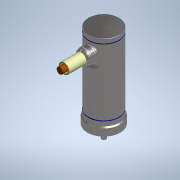
# Autodesk Inventor part: AKMH23x-CCTNCAFK
Saved by Autodesk Inventor 2021 (Build 250183000, 183)
## iProperties
Part Number: AKMH23x-CCTNCAFK
Material: Stainless Steel
Catalog Web Link: www.cadenas.de
Description: AKMH2 Series-AKMH2 Series
Vendor: KOLLMORGEN
Document SubType Name: Modeling
Designer: partserver
Manufacturer: KOLLMORGEN
Mass: 7427.11 g
Surface Area: 696.852 cm^2
Volume: 928.389 cm^3
Density: 8 g/cm^3
Appearance: Semi-Polished
Category: PARTsolutions
Company: KOLLMORGEN
PSOL_IDENT_0: {$CADENAS_DATA\23d-libs\kollmorgen\pilot\akmh2_series.prj},241 {VTYP=3D},{NB=AKMH23x-CCTNCAFK},{LINA=
PSOL_IDENT_1: AKMH23x-CCTNCAFK},{NN=AKMH2 Series},{DATE=23.11.2020 06:56:37},{GEOMDATE=12.11.2020 06:34:38},{VERSI
PSOL_IDENT_2: ON=},{LINEID=20},{WBVAR=ROTORSTACKLENGTH,MOUNT,SHAFT,FEEDBACKDEVICE,CONNECTORS,BRAKE,CL},{WBNUMERIC=
PSOL_IDENT_3: }  {NB=AKMH23x-CCTNCAFK},{LINA=AKMH23x-CCTNCAFK},{KT=DUMMY},{PN=AKMH23x-CCTNCAFK},{SERIES=AKMH2},{RO
PSOL_IDENT_4: TORSTACKLENGTH=3},{MOUNT=C},{SHAFT=C},{SHAFTALG= 'N', 'Smooth shaft [N]', 'C', 'Closed keyway [C]' }
PSOL_IDENT_5: ,{FEEDBACKDEVICE=CA},{CONNECTORS=T},{CONNALG= 'K','Single Cable AKD Connector [K]','T','Single Food
PSOL_IDENT_6: Grade Tubing AKD Connector [T]','V','Single Cable Stainless Vented Connector [V]','W','Single Food G
PSOL_IDENT_7: rade Tubing Stainless Vented Connector [W]','L','Power and Feedback cables terminated with flying le
PSOL_IDENT_8: ads [L]','B','Single Cable Non-Stainless Vented Connector [B]','G','Single Food Grade Tubing Non-Sta
PSOL_IDENT_9: inless Vented Connector [G]', 'P', 'Single SS Straight IP69K Connector [P]' },{BRAKE=N},{CL=F},{SEAL=
PSOL_IDENT_10: K},{D8SKETCH1=205.2},{D2SKETCH1=40},{D1SKETCH2=11},{D4SKETCH2=30},{FACETOFLANGE=U},{M4CLEARANCEHOLE1=
PSOL_IDENT_11: U},{10CLEARANCEHOLE1=S},{M4X07TAPPEDHOLE1=S},{1024TAPPEDHOLE1=S},{CLOSEDKEYWAY=U},{SINGLEHOUSINGFLA=
PSOL_IDENT_12: U},{SINGLECABLEBUSHI=S},{SINGLEFITTINGAND=U},{HYBRIDCABLE=U},{DUALHOUSINGFLAT=S},{DUALCABLEBUSHING=S
PSOL_IDENT_13: },{DUALFITTINGANDTU=S},{FTDHL=C},{FEEDBACKPN=CA},{FL=79},{RPR=0.2-0.7},{CTR=0.3-1.1},{PTR=1.6-5.5},{
PSOL_IDENT_14: MAXS=8000},{MDIA=74},{MC=CC},{C=M4 x 0.7 x 8.0 [.31]},{D=40 (+0.011/-0.005) [1.5748 (+.0004/-.0001)
PSOL_IDENT_15: ] j6},{E=63 [2.480]},{H=D M4 [DIN 332]},{J=11 (+0.012/+0.001) [.4331  (+.0004/+.0001) ] k6},{K=30.0
PSOL_IDENT_16: [1.18]},{P=12.5 (0/-0.13) [.492  (+.000/-.005) ]},{R=4 (0/-0.030)  [.157 (+.0000/-.0010) ]},{S=3.50
PSOL_IDENT_17: [.138]},{T=3.50 [.138]},{U=0.035 [.0013]},{V=0.080 [.0031]},{W=0.080 [.0031]},{ZIN=8.07874},{ZMAX=20
PSOL_IDENT_18: 5.2 [8.079]},{CLALG= '1', '1 meter cable [1]', '2', '2 meter cable [2]', '3'  , '3 meter cable [3]',
PSOL_IDENT_19: '4', '4 meter cable [4]', '5', '5 meter cable [5]'  , '6', '6 meter cable [6]', '7', '7 meter cable
PSOL_IDENT_20: [7]', '8'  , '8 meter cable [8]', '9', '9 meter cable [9]', 'A', '10 meter cable [A]'  , 'B', '11 m
PSOL_IDENT_21: eter cable [B]', 'C', '12 meter cable [C]', 'D'  , '13 meter cable [D]', 'E', '14 meter cable [E]', '
PSOL_IDENT_22: F', '15 meter cable [F]' }
NB: AKMH23x-CCTNCAFK
NN: AKMH2 Series
NT: AKMH2 Series
NBSYN: $PN.
LINA: AKMH23x-CCTNCAFK
CATALOG: Kollmorgen
PN: AKMH23x-CCTNCAFK
SERIES: AKMH2
ROTORSTACKLENGTH: 3
MOUNT: Metric Face [C]
SHAFT: Closed keyway [C]
FEEDBACKDEVICE: Smart feedback device Gen3 [CA]
CONNECTORS: Single Food Grade Tubing AKD Connector [T]
BRAKE: No brake [N]
CL: 15 meter cable [F]
SEAL: K
RPR: 0.2-0.7
CTR: 0.3-1.1
PTR: 1.6-5.5
MAXS: 8000
MDIA: 74
C: M4 x 0.7 x 8.0 [.31]
D: 40 (+0.011/-0.005) [1.5748 (+.0004/-.0001) ] j6
E: 63 [2.480]
H: D M4 [DIN 332]
J: 11 (+0.012/+0.001) [.4331  (+.0004/+.0001) ] k6
K: 30.0 [1.18]
P: 12.5 (0/-0.13) [.492  (+.000/-.005) ]
R: 4 (0/-0.030)  [.157 (+.0000/-.0010) ]
S: 3.50 [.138]
T: 3.50 [.138]
U: 0.035 [.0013]
V: 0.080 [.0031]
W: 0.080 [.0031]
ZMAX: 205.2 [8.079]
SUPPLIER: KOLLMORGEN
ARTICLENO: AKMH23x-CCTNCAFK
BOMINFO: AKMH23x-CCTNCAFK
CREATOR: CADENAS GmbH
Title: AKMH23x-CCTNCAFK
Author: Cadenas PARTsolutions
Comments: AKMH2 Series
Autodesk Inventor part; units mm, degrees
ref_plane "YZ Plane" through (0, 0, 0) normal (1, 0, 0) x (0, 1, 0)
ref_plane "XZ Plane" through (0, 0, 0) normal (0, 1, 0) x (-1, 0, 0)
ref_plane "XY Plane" through (0, 0, 0) normal (0, 0, 1) x (1, 0, 0)
sketch "Sketch1" plane through (0, 0, 0) normal (1, 0, 0) x (0, 0, -1)
  line L0 (207.7, 0) -> (0, 0)
  line L1 (0.5, 0) -> (0.5, 16)
  line L2 (0.5, 16) -> (0, 16.0882)
  line L3 (0, 16.0882) -> (0, 19.5)
  line L4 (0, 19.5) -> (0.5, 20)
  line L5 (0.5, 20) -> (2.5, 20)
  line L6 (2.5, 20) -> (2.5, 39.5)
  line L7 (2.5, 39.5) -> (21, 39.5)
  line L8 (21, 39.5) -> (23.5, 37)
  line L9 (23.5, 37) -> (205.4422, 37)
  arc A0 (206.4416, 36.0349) -> (205.4422, 37) centre (205.4422, 36) ccw
  line L10 (206.4416, 36.0349) -> (207.7, 0)
  line L11 (207.7, 0) -> (0.5, 0)
  constraints: 24 end point, 2 point on circle, 1 centre point
revolve "Revolution1" add sketch "Sketch1" angle 360 about axis through (0, 0, -207.7) along (0, 0, -1)
sketch "Sketch2" plane through (0, 0, 0) normal (1, 0, 0) x (0, 0, -1)
  line L0 (0, 0) -> (-27.5, 0)
  line L1 (-27.5, 0) -> (-27.5, 5)
  line L2 (-27.5, 5) -> (-27, 5.5)
  line L3 (-27, 5.5) -> (-3, 5.5)
  line L4 (-3, 5.5) -> (-3, 7.48)
  line L5 (-3, 7.48) -> (0.5, 7.48)
  line L6 (0.5, 7.48) -> (0.5, 0)
  line L7 (0.5, 0) -> (-27.5, 0)
  constraints: 16 end point
revolve "Revolution2" add sketch "Sketch2" angle 360 about axis through (0, 0, 0) along (0, 0, -1)
sketch "Sketch3" plane through (0, 0, 0) normal (1, 0, 0) x (0, 0, -1)
  line L0 (0.5, 0) -> (-2.5, 0)
  line L1 (-2.5, 7.48) -> (0.5, 7.48)
  line L2 (0.5, 7.48) -> (0.5, 10.1295)
  arc A0 (-2.5, 7.68) -> (0.5, 10.1295) centre (-2, 10.1295) ccw
  line L3 (-2.5, 7.68) -> (-2.5, 7.48)
  constraints: 8 end point, 2 point on circle, 1 centre point
revolve "Revolution3" add sketch "Sketch3" angle 360 about axis through (0, 0, -0.5) along (0, 0, -1)
sketch "Sketch5" plane through (0, 0, 0) normal (1, 0, 0) x (0, 0, -1)
  line L0 (0, 0) -> (-51.7156, 0)
  line L1 (2.5, 39.5) -> (2.5, 37.315)
  line L2 (2.5, 37.315) -> (3.6038, 37.315)
  arc A0 (3.6038, 37.315) -> (4.0989, 37.8846) centre (3.6038, 37.815) ccw
  line L3 (4.0989, 37.8846) -> (3.9, 39.3)
  line L4 (3.9, 39.3) -> (3.9, 39.4)
  arc A1 (4, 39.5) -> (3.9, 39.4) centre (4, 39.4) ccw
  line L5 (4, 39.5) -> (2.5, 39.5)
  constraints: 12 end point, 4 point on circle, 2 centre point
revolve "Revolution4" cut sketch "Sketch5" angle 360 about axis through (0, 0, 0) along (0, 0, -1)
sketch "Sketch6" plane through (0, 0, -2.5) normal (0, 0, 1) x (1, 0, 0)
  point P0 (-22.2739, 22.2739)
hole "Hole1" at (-22.2739, 22.2739, -2.5) direction (0, 0, -1) diameter 3.242 depth 10.1174 tip angle 118 countersink diameter 4 countersink angle 90 thread size "M4x0.7" class "6H" standard "ISO Metric profile"
pattern_linear "Rectangular Pattern1" count 2 spacing 44.5477 along (1, 0, 0) count 2 spacing 44.5477 along (0, -1, 0) of "Hole1"
sketch "Sketch14" plane through (0, 0, 0) normal (1, 0, 0) x (0, 0, -1)
  line L0 (139.6645, -37) -> (193.5355, -37)
  line L1 (193.5355, -37) -> (188.3678, -31.8322)
  arc A0 (188.3678, -31.8322) -> (186.6, -31.1) centre (186.6, -33.6) ccw
  line L2 (186.6, -31.1) -> (146.6, -31.1)
  arc A1 (146.6, -31.1) -> (144.8322, -31.8322) centre (146.6, -33.6) ccw
  line L3 (144.8322, -31.8322) -> (139.6645, -37)
  constraints: 8 end point, 4 point on circle, 2 centre point
extrude "Extrusion1" cut sketch "Sketch14" along normal mid plane 40.0894
sketch "Sketch15" plane through (0, 0, 0) normal (1, 0, 0) x (0, 0, -1)
  arc A0 (-22.5, 2) -> (-22.5, -2) centre (-22.5, 0) ccw
  line L0 (-22.5, -2) -> (-10.5, -2)
  arc A1 (-10.5, -2) -> (-10.5, 2) centre (-10.5, 0) ccw
  line L1 (-10.5, 2) -> (-22.5, 2)
  constraints: 4 end point, 4 point on circle, 2 centre point
extrude "Extrusion2" add sketch "Sketch15" along normal blind 7
sketch "Sketch18" plane through (0, -31.1, 0) normal (0, 1, 0) x (1, 0, 0)
  circle A0 centre (0, 166.6) radius 7.62
  constraints: 1 centre point
extrude "Extrusion3" add sketch "Sketch18" against normal blind 75
sketch "Sketch19" plane through (0, 0, 0) normal (1, 0, 0) x (0, 0, -1)
  line L0 (166.6, -50.4858) -> (166.6, -31.1)
  line L1 (166.6, -31.1) -> (185.6, -31.1)
  line L2 (185.6, -31.1) -> (185.6, -33.7654)
  arc A0 (185.3986, -34.3672) -> (185.6, -33.7654) centre (184.6, -33.7654) ccw
  line L3 (185.3986, -34.3672) -> (185.1041, -34.7581)
  arc A1 (185.1041, -34.7581) -> (184.5, -36.5635) centre (187.5, -36.5635) ccw
  line L4 (184.5, -36.5635) -> (184.5, -44.8599)
  arc A2 (184.391, -45.3139) -> (184.5, -44.8599) centre (183.5, -44.8599) ccw
  line L5 (184.391, -45.3139) -> (183.427, -47.2059)
  arc A3 (183.427, -47.2059) -> (183.1, -48.5679) centre (186.1, -48.5679) ccw
  line L6 (183.1, -48.5679) -> (183.1, -50.4858)
  arc A4 (182.8071, -51.1929) -> (183.1, -50.4858) centre (182.1, -50.4858) ccw
  line L7 (182.8071, -51.1929) -> (179.3, -54.7)
  line L8 (179.3, -54.7) -> (179.3, -96.1)
  line L9 (179.3, -96.1) -> (176.125, -96.1)
  line L10 (176.125, -96.1) -> (176.125, -50.4858)
  line L11 (176.125, -50.4858) -> (166.6, -50.4858)
  line L12 (166.6, -50.4858) -> (166.6, -31.1)
  constraints: 26 end point, 10 point on circle, 5 centre point
revolve "Revolution5" add sketch "Sketch19" angle 360 about axis through (0, -50.4858, -166.6) along (0, -1, 0)
sketch "Sketch20" plane through (0, 0, 0) normal (1, 0, 0) x (0, 0, -1)
  line L0 (193.6472, 0) -> (0, 0)
  line L1 (34, 37) -> (35.7, 37)
  arc A0 (35.7, 37) -> (34, 37) centre (34.85, 35.3238) ccw
  constraints: 4 end point, 2 point on circle, 1 centre point
revolve "Revolution6" add sketch "Sketch20" angle 360 about axis through (0, 0, -193.6472) along (0, 0, -1)
sketch "Sketch_1" plane through (0, 0, 0) normal (1, 0, 0) x (0, 0, -1)
  line L0 (193.6472, 0) -> (0, 0)
  line L1 (194.86, 37) -> (196.56, 37)
  arc A0 (196.56, 37) -> (194.86, 37) centre (195.71, 35.3238) ccw
  constraints: 4 end point, 2 point on circle, 1 centre point
revolve "Revolution7" add sketch "Sketch_1" angle 360 about axis through (0, 0, -193.6472) along (0, 0, -1)
body "Solid1"
